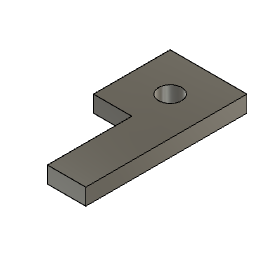
x_gantry_belt_pretensioner (Autodesk Fusion 360 design; units mm, degrees)
Autodesk Fusion 360 part; units mm, degrees
sketch "Sketch1" plane through (0, 0, 0) normal (0, 0, 1) x (1, 0, 0) in component "pretensioner"
  line L0 (10, 0) -> (20, 0)
  line L1 (20, 0) -> (20, 42)
  line L2 (20, 42) -> (0, 42)
  line L3 (0, 42) -> (0, 22)
  line L4 (0, 42) -> (20, 42) construction
  line L5 (20, 42) -> (20, 22) construction
  line L6 (20, 22) -> (0, 22) construction
  line L7 (0, 22) -> (0, 42) construction
  circle A0 centre (10, 32) radius 3
  line L8 (10, 22) -> (10, 0)
  line L9 (10, 0) -> (20, 0)
  line L10 (20, 0) -> (20, 22)
  line L11 (10, 22) -> (0, 22)
  dimension "d1" = 20
  dimension "d2" = 42
  dimension "d3" = 20
  dimension "d4" = 6
  dimension "d5" = 10
  constraint horizontal L0
  constraint vertical L1
  constraint horizontal L2
  constraint vertical L3
  constraint horizontal L4
  constraint vertical L5
  constraint horizontal L6
  constraint vertical L7
  constraint vertical L8
  constraint horizontal L9
  constraint vertical L10
  measures "d1" distance of origin L0.end
  measures "d2" distance of origin L2.end
  measures "d3" distance of L2.end L3.end
  measures "d4" diameter of A0
  measures "d5" distance of L5.end L8.start
extrude "Extrude1" add sketch "Sketch1" along normal blind 4.3 in component "pretensioner"
component "pretensioner" placed x (1, 0, 0) y (0, 1, 0) z (0, 0, 1) at (0, 0, 0)
